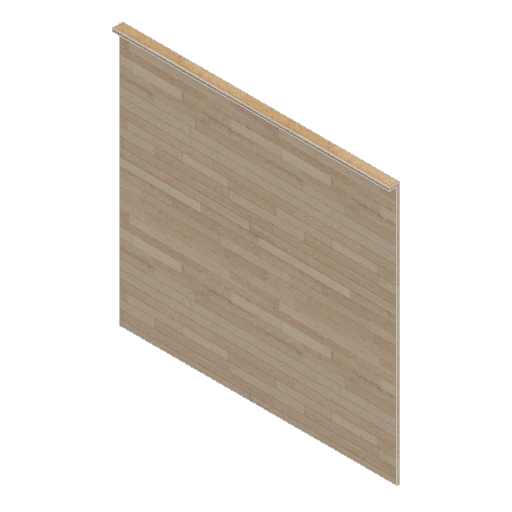
# Autodesk Inventor part: blat
Saved by Autodesk Inventor 2025.1 (Build 291241000, 241)
## iProperties
Created: 2023-06-13
Part Number: blat
Material: Drewno (klon)
Document SubType Name: Modeling
Designer: MateuszWawrzyniak
Density: 0.67 g/cm^3
Appearance: Klon naturalny — lśniący — ciemny odcień
Author: MateuszWawrzyniak
Autodesk Inventor part; units mm, degrees
ref_plane "YZ Plane" through (0, 0, 0) normal (1, 0, 0) x (0, 1, 0)
ref_plane "XZ Plane" through (0, 0, 0) normal (0, 1, 0) x (-1, 0, 0)
ref_plane "XY Plane" through (0, 0, 0) normal (0, 0, 1) x (1, 0, 0)
sketch "Szkic1" plane through (0, 0, 0) normal (0, 0, 1) x (1, 0, 0)
  line L0 (0, 0) -> (1800, 0)
  line L1 (1800, 0) -> (1800, 1700)
  line L2 (1800, 1700) -> (0, 1700)
  line L3 (0, 1700) -> (0, 0)
  line L4 (0, 1681) -> (1800, 1681)
  dimension "d0" = 1800
  dimension "d1" = 1700
  dimension "d2" = 19
  constraints: 10 end point, 2 parallel, 2 perpendicular, 2 point on line, 1 horizontal
  measures "d0" distance of L2.end L1.end
  measures "d1" distance of L1.end L0.end
  measures "d2" distance between parallel lines of L2 L4
extrude "Wyciągnięcie proste1" add sketch "Szkic1" along normal blind 69 contours L3 L2 L1 L4
extrude "Wyciągnięcie proste2" add sketch "Szkic1" along normal blind 19 contours L3 L4 L1 L0
